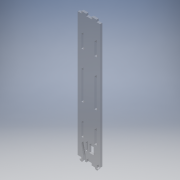
# Autodesk Inventor part: Left_wall
Saved by Autodesk Inventor 2016 (Build 200138000, 138)
## iProperties
Created: 2015-06-19
Part Number: Left_wall
Material: Generic
Document SubType Name: Modeling
Designer: Openlab
Density: 1 g/cm^3
Appearance: Polycarbonate - Clear
Author: Openlab
Autodesk Inventor part; units mm, degrees
ref_plane "YZ Plane" through (0, 0, 0) normal (1, 0, 0) x (0, 1, 0)
ref_plane "XZ Plane" through (0, 0, 0) normal (0, 1, 0) x (-1, 0, 0)
ref_plane "XY Plane" through (0, 0, 0) normal (0, 0, 1) x (1, 0, 0)
sketch "Sketch1" plane through (0, 0, 0) normal (0, 1, 0) x (-1, 0, 0)
  line L0 (26.5, -25) -> (23.5, -25)
  line L1 (26.5, -43) -> (23.5, -43)
  line L2 (26.5, -68) -> (23.5, -68)
  line L3 (26.5, -108) -> (23.5, -108)
  line L4 (8, -68) -> (5, -68)
  line L5 (8, -108) -> (5, -108)
  line L6 (8, -43) -> (5, -43)
  line L7 (8, -25) -> (5, -25)
  line L8 (23.5, -108) -> (23.5, -68)
  line L9 (23.5, -43) -> (23.5, -25)
  line L10 (8, -108) -> (8, -68)
  line L11 (8, -43) -> (8, -25)
  line L12 (8, -151) -> (8, -133)
  line L13 (26.5, -133) -> (23.5, -133)
  line L14 (8, -133) -> (5, -133)
  line L15 (23.5, -133) -> (23.5, -151)
  line L16 (23.5, -151) -> (26.5, -151)
  line L17 (5, -151) -> (8, -151)
  line L18 (20.5, -155.0739) -> (18.7, -155.0739)
  line L19 (18.7, -155.0739) -> (18.7, -165.0739)
  line L20 (18.7, -165.0739) -> (20.5, -165.0739)
  line L21 (20.5, -165.0739) -> (20.5, -155.0739)
  line L22 (5, -176) -> (0, -176)
  line L23 (15.75, -82) -> (15.75, -115) construction
  line L24 (15.2, -155.0739) -> (9.2, -155.0739)
  line L25 (9.2, -155.0739) -> (9.2, -165.0739)
  line L26 (9.2, -165.0739) -> (15.2, -165.0739)
  line L27 (15.2, -165.0739) -> (15.2, -155.0739)
  line L28 (26.5, -25) -> (26.5, -43)
  line L29 (26.5, -68) -> (26.5, -108)
  line L30 (26.5, -133) -> (26.5, -151)
  line L31 (5, -151) -> (5, -133)
  line L32 (5, -108) -> (5, -68)
  line L33 (5, -43) -> (5, -25)
  line L34 (31.5, 0) -> (31.5, -176)
  line L35 (0, -176) -> (0, 0)
  line L36 (5, 0) -> (0, 0)
  line L37 (26.5, 0) -> (26.5, 3)
  line L38 (26.5, 3) -> (19.5, 3)
  line L39 (19.5, 3) -> (19.5, 0)
  line L40 (19.5, 0) -> (12, 0)
  line L41 (12, 0) -> (12, 3)
  line L42 (12, 3) -> (5, 3)
  line L43 (5, 3) -> (5, 0)
  line L44 (26.5, 0) -> (31.5, 0)
  line L45 (5, -176) -> (5, -179)
  line L46 (7.5, -179) -> (12, -179)
  line L47 (12, -179) -> (12, -176)
  line L48 (12, -176) -> (19.5, -176)
  line L49 (19.5, -176) -> (19.5, -179)
  line L50 (19.5, -179) -> (21.5, -179)
  line L51 (26.5, -179) -> (26.5, -176)
  line L52 (26.5, -176) -> (31.5, -176)
  arc A0 (24, -179) -> (29, -179) centre (26.5, -179) ccw
  line L53 (26.5, -179) -> (29, -179)
  arc A1 (2.5, -179) -> (7.5, -179) centre (5, -179) ccw
  line L54 (5, -179) -> (2.5, -179)
  line L55 (24, -179) -> (24, -172.2262)
  line L56 (24, -172.2262) -> (26.6099, -158.5778)
  line L57 (25.4256, -158.2886) -> (21.5, -171.441)
  line L58 (21.5, -171.441) -> (21.5, -179)
  arc A2 (26.6099, -158.5778) -> (25.4256, -158.2886) centre (26.0105, -158.4632) ccw
  dimension "d7" = 18
  dimension "d8" = 25
  dimension "d9" = 40
  dimension "d39" = 18
  dimension "d43" = 1.8
  dimension "d45" = 10
  dimension "d46" = 3
  dimension "d51" = 3.5
  dimension "d52" = 6
  dimension "d55" = 5
  dimension "d56" = 3
  dimension "d60" = 10.9261
  dimension "d61" = 25
  dimension "d62" = 15.5
  dimension "d63" = 25
  dimension "d64" = 25
  dimension "d65" = 7
  dimension "d66" = 5
  dimension "d68" = 7
  dimension "d69" = 7
  dimension "d70" = 2.5
  dimension "d73" = 5
  dimension "d74" = 176
  constraints: 119 end point, 23 collinear, 16 perpendicular, 8 point on line, 7 equal length, 7 vertical, 6 point on circle, 5 horizontal, 5 parallel, 3 centre point, 2 coincident, 2 tangent, 1 equal radius, 5 other
  measures "d7" distance between parallel lines of L1 L0
  measures "d8" distance between parallel lines of L2 L1
  measures "d9" distance between parallel lines of L3 L2
  measures "d39" distance of L13.end L15.end
  measures "d43" distance of L18.start L18.end
  measures "d45" distance of L20.end L18.start
  measures "d46" distance between parallel lines of L21 L15
  measures "d51" distance between parallel lines of L19 L27
  measures "d52" distance of L24.start L24.end
  measures "d55" distance between parallel lines of L35 L31
  measures "d56" distance of L0.start L0.end
  measures "d60" distance between parallel lines of L22 L26
  measures "d61" distance between parallel lines of L3 L13
  measures "d62" distance between parallel lines of L10 L8
  measures "d63" distance between parallel lines of L44 L0
  measures "d64" distance between parallel lines of L16 L52
  measures "d65" distance of L37.end L38.end
  measures "d66" diameter of A0
  measures "d68" distance between parallel lines of L49 L51
  measures "d69" distance between parallel lines of L45 L47
  measures "d70" distance between parallel lines of L58 L55
  measures "d73" distance of L22.start L22.end
  measures "d74" distance between parallel lines of L52 L44
extrude "Extrusion3" add sketch "Sketch1" along normal blind 3
body "Solid3"
